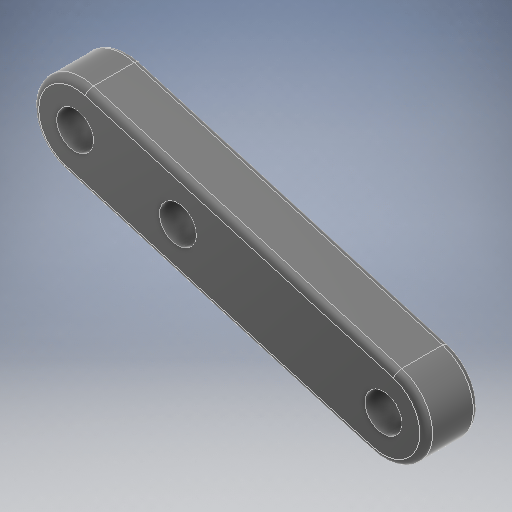
# Autodesk Inventor part: RigidPieceFloat
Saved by Autodesk Inventor 2026.1 (Build 301233000, 233)
## iProperties
Created: 2025-09-29
Part Number: RigidPieceFloat
Material: Plastic, Opaque Black
Document SubType Name: Modeling
Designer: Teddy
Density: 0.952 g/cm^3
Appearance: Smooth - Black
Author: Teddy
Autodesk Inventor part; units mm, degrees
ref_plane "YZ Plane" through (0, 0, 0) normal (1, 0, 0) x (0, 1, 0)
ref_plane "XZ Plane" through (0, 0, 0) normal (0, 1, 0) x (-1, 0, 0)
ref_plane "Work Plane1" through (98.0034, 4.8347, 0) normal (0, 0, -1) x (-0.9323, -0.3616, 0)
sketch "Sketch1" plane through (98.0034, 4.8347, 0) normal (0, 0, -1) x (-0.9323, -0.3616, 0)
  circle A0 centre (1.1498, 63.5) radius 2.1844 projected
  circle A1 centre (21.2874, 78.9802) radius 2.1844
  circle A2 centre (31.3562, 86.7203) radius 2.1844 projected
  line L0 (1.1498, 63.5) -> (1.1498, 86.7203) construction
  line L1 (4.2458, 59.4725) -> (34.4523, 82.6927)
  line L2 (28.2602, 90.7478) -> (-1.9463, 67.5275)
  arc A3 (-1.9463, 67.5275) -> (4.2458, 59.4725) centre (1.1498, 63.5) ccw
  arc A4 (34.4523, 82.6927) -> (28.2602, 90.7478) centre (31.3562, 86.7203) ccw
  point P0 (93.1204, 30.9293)
  point P1 (1.1498, 94.7574)
  dimension "d0" = 10.16
  dimension "d4" = 12.7
  constraints: 8 end point, 4 point on circle, 4 tangent, 3 centre point, 1 parallel, 1 point on line, 1 vertical
  measures "d0" diameter of A4
  measures "d4" distance of L0.end A1.centre
extrude "Extrusion1" add sketch "Sketch1" along normal blind 6.35
fillet "Fillet1" radius 0.762 8 edges at (32.5372, 75.7795, -6.35) (57.1214, 73.8604, -6.35) (78.845, 62.1922, -6.35) (54.2609, 64.1113, -6.35) (78.845, 62.1922, 0) (54.2609, 64.1113, 0) (32.5372, 75.7795, 0) (57.1214, 73.8604, 0)
body "Solid1"
